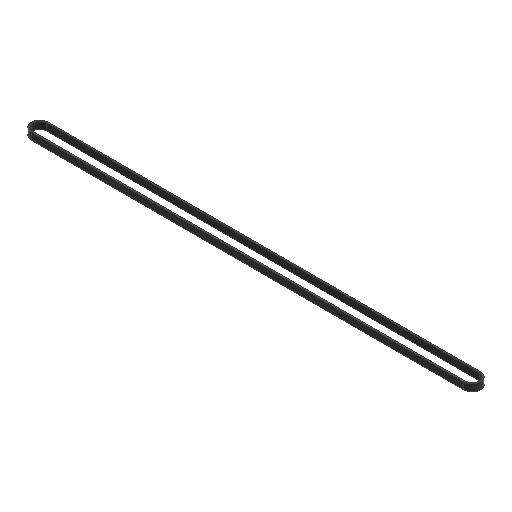
# Autodesk Inventor part: COTS_GENERIC_X_Axis_Timing_Belt
Saved by Autodesk Inventor 2026.1 (Build 301233000, 233)
## iProperties
Created: 2017-05-29
Part Number: COTS_GENERIC_X_Axis_Timing_Belt
Material: Ogólny
Document SubType Name: Modeling
Designer: Andrzej
Density: 1 g/cm^3
Appearance: Gładkie - czarne
Mass: 7.40378 g
Surface Area: 129.272 cm^2
Volume: 7.40378 cm^3
Author: Andrzej
Autodesk Inventor part; units mm, degrees
ref_plane "YZ Plane" through (0, 0, 0) normal (1, 0, 0) x (0, 1, 0)
ref_plane "XZ Plane" through (0, 0, 0) normal (0, 1, 0) x (-1, 0, 0)
ref_plane "XY Plane" through (0, 0, 0) normal (0, 0, 1) x (1, 0, 0)
sketch "Szkic1" plane through (0, 0, 0) normal (0, 0, 1) x (1, 0, 0)
  line L0 (-211.8041, 0) -> (185.2919, 0) construction
  line L1 (-211.8041, -6.5) -> (185.2919, -6.5)
  line L2 (185.2919, 6.5) -> (-211.8041, 6.5)
  arc A0 (-211.8041, 6.5) -> (-211.8041, -6.5) centre (-211.8041, 0) ccw
  arc A1 (185.2919, -6.5) -> (185.2919, 6.5) centre (185.2919, 0) ccw
  line L3 (-211.8041, 7.9) -> (185.2919, 7.9)
  arc A2 (185.2919, -7.9) -> (185.2919, 7.9) centre (185.2919, 0) ccw
  line L4 (185.2919, -7.9) -> (-211.8041, -7.9)
  arc A3 (-211.8041, 7.9) -> (-211.8041, -7.9) centre (-211.8041, 0) ccw
  point P0 (0, 0)
  point P1 (-13.2561, 0)
  dimension "d0" = 198.548
  dimension "d1" = 13
  dimension "d2" = 1.4
  constraints: 12 end point, 8 point on circle, 4 centre point, 4 tangent, 2 parallel, 1 horizontal, 1 midpoint, 3 other
  measures "d0" distance of point (-13.256, 0) L0.end
  measures "d1" diameter of A1
  measures "d2" distance between parallel lines of L2 L3
extrude "Wyciągnięcie proste1" add sketch "Szkic1" along normal blind 6.3
